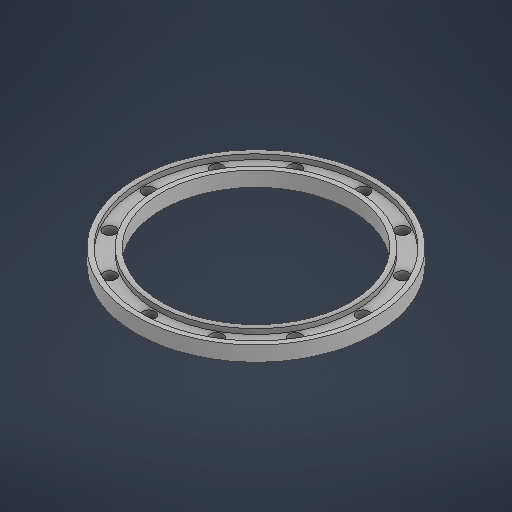
# Autodesk Inventor part: P_magnetCase
Saved by Autodesk Inventor 2026 (Build 300175000, 175)
## iProperties
Created: 2025-05-06
Part Number: P_magnetCase
Material: ABS-Kunststoff
Document SubType Name: Modeling
Designer: FAL
Density: 1.06 g/cm^3
Appearance: Hellgrau
Author: FAL
Autodesk Inventor part; units mm, degrees
ref_plane "YZ Plane" through (0, 0, 0) normal (1, 0, 0) x (0, 1, 0)
ref_plane "XZ Plane" through (0, 0, 0) normal (0, 1, 0) x (-1, 0, 0)
ref_plane "XY Plane" through (0, 0, 0) normal (0, 0, 1) x (1, 0, 0)
sketch "Skizze1" plane through (0, 0, 0) normal (0, 0, 1) x (1, 0, 0)
  circle A0 centre (0, 0) radius 38
  circle A1 centre (0, 0) radius 48
  dimension "d0" = 76
  dimension "d1" = 10
  constraints: 2 centre point, 2 coincident
  measures "d0" diameter of A0
  measures "d1" radial gap between concentric circles of A1 A0
extrude "Extrusion1" add sketch "Skizze1" along normal blind 6
sketch "Skizze3" plane through (0, 0, 6) normal (0, 0, 1) x (1, 0, 0)
  circle A0 centre (0, 0) radius 40
  circle A1 centre (0, 0) radius 46
  circle A2 centre (0, 0) radius 38 projected
  circle A3 centre (0, 0) radius 48 projected
  dimension "d8" = 2
  dimension "d9" = 2
  constraints: 2 centre point, 2 coincident
  measures "d8" radial gap between concentric circles of A2 A0
  measures "d9" radial gap between concentric circles of A3 A1
extrude "Extrusion3" cut sketch "Skizze3" against normal blind 2 contours A1
sketch "Skizze5" plane through (0, 0, 4) normal (0, 0, 1) x (1, 0, 0)
  circle A0 centre (0, 0) radius 46 projected
  line L0 (0, 46) -> (0, 40)
  circle A1 centre (0, 0) radius 40 projected
  circle A2 centre (0, 43) radius 2.5
  dimension "d12" = 5
  constraints: 2 end point, 2 vertical alignment, 1 centre point, 1 midpoint, 1 vertical, 2 other
  measures "d12" diameter of A2
extrude "Extrusion4" cut sketch "Skizze5" against normal blind 4 contours A2 L0 | L0 A2
pattern_circular "Runde Anordnung1" count 12 over 360 about axis through (0, 0, -10) along (0, 0, 1) of "Extrusion4"
